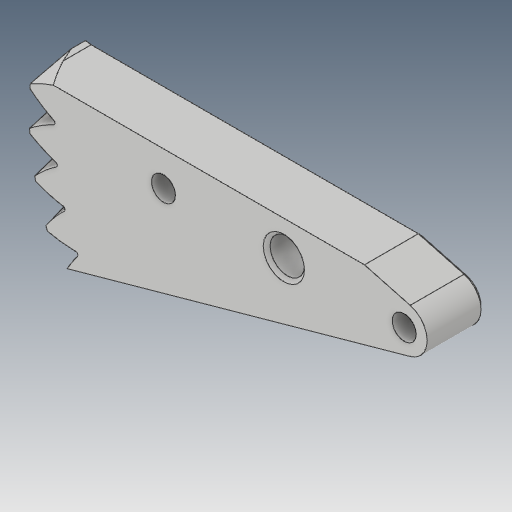
# Autodesk Inventor part: tilt-gear_C
Saved by Autodesk Inventor 2018 (Build 220112000, 112)
## iProperties
Created: 2019-02-22
Part Number: tilt-gear_C
Material: Generic
Document SubType Name: Modeling
Designer: Tsche
Density: 1 g/cm^3
Appearance: Default
Author: Tsche
Autodesk Inventor part; units mm, degrees
ref_plane "YZ Plane" through (0, 0, 0) normal (1, 0, 0) x (0, 1, 0)
ref_plane "XZ Plane" through (0, 0, 0) normal (0, 1, 0) x (-1, 0, 0)
ref_plane "XY Plane" through (0, 0, 0) normal (0, 0, 1) x (1, 0, 0)
sketch "Block1" plane through (0, 0, 0) normal (0, 0, 1) x (1, 0, 0)
  spline S0 degree 3 poles (-1.5139, 22.1715) (-1.4436, 22.0829) (-1.3029, 21.9057) (-1.1015, 21.6325) (-0.9075, 21.3539) (-0.7222, 21.0696) (-0.546, 20.7794) (-0.3796, 20.4835) (-0.2635, 20.257) (-0.1951, 20.1173) (-0.1716, 20.0658) (-0.1498, 20.0293) (-0.1267, 20.0021) (-0.1041, 19.985) (-0.0784, 19.9725) (-0.0422, 19.9718) (0, 19.9739) (0.0422, 19.9718) (0.0784, 19.9725) (0.1041, 19.985) (0.1267, 20.0021) (0.1498, 20.0293) (0.1716, 20.0658) (0.1951, 20.1173) (0.2635, 20.257) (0.3796, 20.4835) (0.546, 20.7794) (0.7222, 21.0696) (0.9075, 21.3539) (1.1015, 21.6325) (1.3029, 21.9057) (1.4436, 22.0829) (1.5139, 22.1715) knots 0 0 0 0 0.033938 0.067876 0.101814 0.135752 0.16969 0.203627 0.237565 0.246049 0.250292 0.254532 0.258768 0.260888 0.263008 0.267236 0.271483 0.27573 0.279957 0.282078 0.284198 0.288434 0.292674 0.296917 0.305401 0.339339 0.373276 0.407214 0.441152 0.47509 0.509028 0.542966 0.542966 0.542966 0.542966
  circle A0 centre (0, 0) radius 19.9732 construction
  circle A1 centre (0, 0) radius 18.217 construction
  circle A2 centre (0, 0) radius 21.2232 construction
  circle A3 centre (0, 0) radius 22.2232 construction
  arc A4 (1.5139, 22.1715) -> (-1.5139, 22.1715) centre (0, 0) ccw
  line L0 (0, 22.2232) -> (0, 19.9732) construction
  point P0 (0, 18.3765)
  point P1 (-1.3045, 21.9044)
  point P2 (-1.1027, 21.6316)
  point P3 (-0.9089, 21.353)
  point P4 (-0.7237, 21.0686)
  point P5 (-0.5477, 20.7784)
  point P6 (-0.3816, 20.4825)
  point P7 (-0.2263, 20.1807)
  point P8 (-0.1893, 20.1043)
  point P9 (-0.1709, 20.0661)
  point P10 (-0.1488, 20.0299)
  point P11 (-0.1207, 19.9982)
  point P12 (-0.1037, 19.9856)
  point P13 (-0.0845, 19.9766)
  point P14 (-0.0425, 19.9723)
  point P15 (0.0425, 19.9723)
  point P16 (0.0845, 19.9766)
  point P17 (0.1037, 19.9856)
  point P18 (0.1207, 19.9982)
  point P19 (0.1488, 20.0299)
  point P20 (0.1709, 20.0661)
  point P21 (0.1893, 20.1043)
  point P22 (0.2263, 20.1807)
  point P23 (0.3816, 20.4825)
  point P24 (0.5477, 20.7784)
  point P25 (0.7237, 21.0686)
  point P26 (0.9089, 21.353)
  point P27 (1.1027, 21.6316)
  point P28 (1.3045, 21.9044)
sketch "Sketch1" plane through (0, 0, 0) normal (0, 0, 1) x (1, 0, 0)
  line L0 (0, -13.3863) -> (0, 5.8125) construction
  line L1 (-30.1989, 0) -> (19.6272, 0) construction
  arc A0 (-22.01, 3.0698) -> (-19.6108, -10.4536) centre (0, 0) ccw
  line L2 (-19.6108, -10.4536) -> (0, 0) construction
  line L3 (0, 0) -> (-22.01, 3.0698) construction
  line L4 (-21.8813, -3.8819) -> (0, 0) construction
  arc A1 (-21.0195, 2.9317) -> (-18.7284, -9.9832) centre (0, 0) ccw construction
  circle A2 centre (-10.5, 0) radius 1.05
  circle A3 centre (10.5, 0) radius 1.05
  line L5 (-21.5095, 3) -> (7.0313, 3)
  arc A4 (11.0361, -1.9268) -> (11.0176, 1.9319) centre (10.5, 0) ccw
  line L6 (-19.6108, -10.4536) -> (11.0361, -1.9268)
  line L7 (-22.01, 3.0698) -> (-21.5095, 3)
  line L8 (11.0176, 1.9319) -> (7.0313, 3)
  circle A5 centre (0, 0) radius 1.5
  dimension "d0" = 18
  dimension "d1" = 10.06
  dimension "d2" = 1
  dimension "d3" = 21.223
  dimension "d4" = 2.1
  dimension "d5" = 21
  dimension "d6" = 2
  dimension "d40" = 3
  dimension "d41" = 15
  dimension "d42" = 3
  constraints: 14 end point, 7 point on circle, 6 centre point, 4 point on line, 3 coincident, 2 tangent, 1 concentric, 1 perpendicular, 1 symmetric about line, 1 other
  measures "d0" angle of L3 L4
  measures "d1" angle of L1 L4
  measures "d2" radial gap between concentric circles of A1 A0
  measures "d3" radius of A1
  measures "d4" diameter of A2
  measures "d5" distance of A3.centre A2.centre
  measures "d6" radius of A4
  measures "d40" distance between parallel lines of L5 L1
  measures "d41" angle of L5 L8
  measures "d42" diameter of A5
extrude "Extrusion1" add sketch "Sketch1" along normal blind 5
chamfer "Chamfer3" distance 0.3 angle 45 5 edges at (-7.2391, 3, 0) (9.0244, 2.4659, 0) (12.5, 0.0096, 0) (-4.2874, -6.1902, 0) (-21.7597, 3.0349, 0)
sketch "Sketch2" plane through (0, 0, 5) normal (0, 0, 1) x (1, 0, 0)
  line L0 (-33.1271, 0) -> (33.1271, 0) construction
  spline S0 degree 3 poles (22.0203, 2.996) (21.9366, 2.9199) (21.7691, 2.7677) (21.51, 2.5484) (21.2452, 2.3362) (20.9738, 2.1322) (20.6961, 1.937) (20.4121, 1.7512) (20.1938, 1.6201) (20.059, 1.5425) (20.0092, 1.5156) (19.9743, 1.4914) (19.9487, 1.4666) (19.9331, 1.4429) (19.9224, 1.4164) (19.9241, 1.3802) (19.929, 1.3383) (19.9297, 1.296) (19.9329, 1.26) (19.9471, 1.2351) (19.9656, 1.2137) (19.9944, 1.1925) (20.0322, 1.1732) (20.0851, 1.1532) (20.2291, 1.0944) (20.4629, 0.9936) (20.7693, 0.8474) (21.0706, 0.6911) (21.3668, 0.5253) (21.6576, 0.3504) (21.9437, 0.1677) (22.13, 0.0392) (22.2231, -0.025) knots 0 0 0 0 0.033938 0.067876 0.101814 0.135752 0.16969 0.203627 0.237565 0.246049 0.250292 0.254532 0.258768 0.260888 0.263008 0.267236 0.271483 0.27573 0.279957 0.282078 0.284198 0.288434 0.292674 0.296917 0.305401 0.339339 0.373276 0.407214 0.441152 0.47509 0.509028 0.542966 0.542966 0.542966 0.542966
  circle A0 centre (0, 0) radius 19.9732 construction
  circle A1 centre (0, 0) radius 18.217 construction
  circle A2 centre (0, 0) radius 21.2232 construction
  circle A3 centre (0, 0) radius 22.2232 construction
  arc A4 (22.2231, -0.025) -> (22.0203, 2.996) centre (0, 0) ccw
  line L1 (22.1732, 1.489) -> (19.9283, 1.3382) construction
  point P0 (0, 0)
  point P1 (0, 0)
  dimension "d28" = 183.842
  constraints: 2 other
coil "Coil1" sketch "Sketch2" operation cut axis through (0, 0, -10) along (0, 0, -1) pitch 497.6617 turns 0.010047 hand right
pattern_circular "Circular Pattern1" count 41 over 360 about axis through (0, 0, -10) along (0, 0, 1) of "Coil1"
chamfer "Chamfer2" distance 0.3 angle 45 9 edges at (9.45, 0, 0) (-11.55, 0, 0) (-20.1231, 1.2486, 0) (-19.9084, -1.6071, 0) (-19.4298, -4.6272, 0) (-18.4957, -7.5389, 0) (-1.5, 0, 0) (-1.5, 0, 5) (-19.6863, -10.1203, 0)
equation "\"d42\" = bore_press"
equation "\"d43\" = champfer"
equation "\"d37\" = champfer"
equation "\"finger_width\" = 25"
equation "\"finger_thickness\" = 8"
equation "\"finger_part_A_length\" = 42.8625"
equation "\"finger_part_B_length\" = 28.575"
equation "\"finger_link_width\" = 3.5"
equation "\"finger_link_clearence\" = 0.15"
equation "\"tol\" = 0.5 * finger_link_clearence"
equation "\"link_tol\" = 0.254"
equation "\"bore_press\" = 3"
equation "\"bore_clearance\" = 3.1"
equation "\"bar_diameter\" = 6.5"
equation "\"bar_thickness\" = 4"
equation "\"bar_width\" = 7"
equation "\"hinge_dist_sym_plane\" = 4"
equation "\"hinge_thickness\" = 3"
equation "\"hinge_act_length_c\" = 7.62"
equation "\"hinge_act_length_bc\" = 16.66875"
equation "\"hinge_act_length_ab\" = 11.049"
equation "\"hinge_act_length_a\" = 21.43125"
equation "\"hinge_guid_length_c\" = 9.525"
equation "\"hinge_guid_length_bc\" = 9.525"
equation "\"hinge_guid_length_ab\" = 17.145"
equation "\"hinge_guid_length_a\" = 17.145"
equation "\"bar_length_bc\" = finger_part_B_length"
equation "\"bar_act_length_ab\" = 40.48125"
equation "\"bar_guid_length_ab\" = 43.275"
equation "\"champfer\" = 0.3"
equation "\"fillet\" = 0.4"
equation "\"dist_finger_BC\" = 56.5"
equation "\"gear_diameter\" = 14"
equation "\"hinge_point\" = 16.5"
equation "\"dist_hinge_points\" = 56.5"
body "Solid1"
